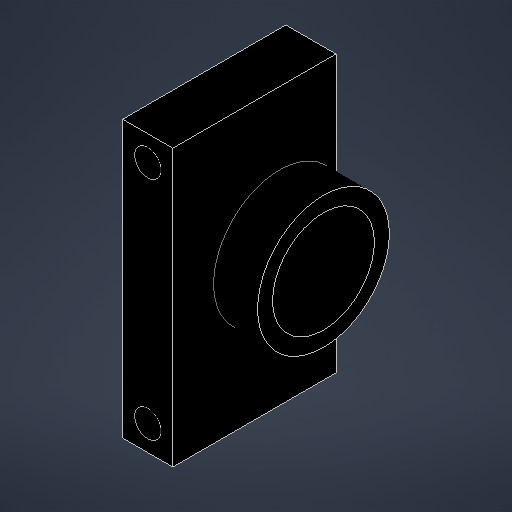
# Autodesk Inventor part: Motor Bracket
Saved by Autodesk Inventor 2026.1 (Build 301233020, 233B)
## iProperties
Created: 2025-11-06
Part Number: Motor Bracket
Material: Generic
Document SubType Name: Modeling
Designer: Bahaa
Density: 1 g/cm^3
Appearance: Black PLA
Mass: 8.44475 g
Surface Area: 48.2722 cm^2
Volume: 8.44475 cm^3
Author: Bahaa
Autodesk Inventor part; units mm, degrees
ref_plane "YZ Plane" through (0, 0, 0) normal (1, 0, 0) x (0, 1, 0)
ref_plane "XZ Plane" through (0, 0, 0) normal (0, 1, 0) x (-1, 0, 0)
sketch "Sketch1" plane through (0, 0, 0) normal (0, 1, 0) x (-1, 0, 0)
  line L0 (4, 22) -> (-4, 22)
  line L1 (-4, 22) -> (-4, -22)
  line L2 (-4, -22) -> (4, -22)
  line L3 (4, -22) -> (4, 22)
  line L4 (4, 22) -> (-4, -22) construction
  line L5 (-4, 22) -> (4, -22) construction
  point P0 (0, 0)
  dimension "d0" = 8
  dimension "d1" = 44
  constraints: 12 end point, 2 midpoint, 2 parallel, 1 horizontal, 1 perpendicular
  measures "d0" distance of L2.end L1.end
  measures "d1" distance of L1.end L0.end
extrude "Extrusion1" add sketch "Sketch1" along normal blind 26
sketch "Sketch2" plane through (4, 0, 22) normal (1, 0, 0) x (0, 0, -1)
  circle A0 centre (22, 17) radius 8.1
  line L0 (0, 0) -> (0, 26) projected
  line L1 (44, 0) -> (44, 26) projected
  line L2 (0, 0) -> (44, 0) projected
  line L3 (0, 26) -> (44, 26) projected
  circle A1 centre (22, 17) radius 4.1
  circle A2 centre (22, 17) radius 5.1
  circle A3 centre (22, 17) radius 28 construction
  circle A4 centre (22, 17) radius 10.5
  line L4 (17.7, 21.3) -> (26.3, 21.3)
  line L5 (26.3, 21.3) -> (26.3, 12.7)
  line L6 (26.3, 12.7) -> (17.7, 12.7)
  line L7 (17.7, 12.7) -> (17.7, 21.3)
  line L8 (17.7, 21.3) -> (26.3, 12.7) construction
  line L9 (26.3, 21.3) -> (17.7, 12.7) construction
  point P0 (22, 0)
  point P1 (34.4721, 0)
  point P2 (25.5279, 0)
  dimension "d4" = 16.2
  dimension "d5" = 44
  dimension "d6" = 26
  dimension "d7" = 17
  dimension "d8" = 22
  dimension "d12" = 8.2
  dimension "d15" = 10.2
  dimension "d20" = 56
  dimension "d27" = 21
  dimension "d53" = 8.6
  dimension "d54" = 8.6
  constraints: 12 end point, 5 centre point, 4 coincident, 2 midpoint, 2 parallel, 1 horizontal, 1 perpendicular
  measures "d4" diameter of A0
  measures "d5" distance between parallel lines of L0 L1
  measures "d6" distance between parallel lines of L2 L3
  measures "d7" distance from line of L2 A0.centre
  measures "d8" distance from line of L1 A0.centre
  measures "d12" diameter of A1
  measures "d15" diameter of A2
  measures "d20" diameter of A3
  measures "d27" diameter of A4
  measures "d53" distance of L5.end L6.end
  measures "d54" distance of L4.end L5.end
sketch "Sketch3" plane through (0, 26, 0) normal (0, 1, 0) x (1, 0, 0)
  line L0 (4, -22) -> (4, 22) projected
  line L1 (-4, 22) -> (-4, -22) projected
  line L2 (-4, -22) -> (4, -22) projected
  line L3 (4, 0) -> (-4, 0) construction
  point P0 (0, 0)
  point P1 (0, -18)
  point P2 (0, 18)
  dimension "d9" = 8
  dimension "d18" = 4
  dimension "d19" = 4
  constraints: 2 end point, 2 midpoint, 1 symmetric about line
  measures "d9" distance between parallel lines of L0 L1
  measures "d18" distance from line of L2 point (0, -18)
  measures "d19" distance from line of L0 point (0, -18)
extrude "Extrusion2" cut sketch "Sketch2" against normal blind 5 contours A0 | A1 | A2 L5 | L5 A2 L6 L7 L4 | A2 L4 L5 | L5 L6 A2 | L4 A2 | A2 L6 | A2 L7 L4 | L6 L7 A2 | L7 A2
extrude "Extrusion3" cut sketch "Sketch2" against normal through all contours A1 | L5 A2 L6 L7 L4 | A2 L4 L5 | L5 L6 A2 | A2 L7 L4 | L6 L7 A2
extrude "Extrusion4" cut sketch "Sketch2" against normal blind 1.15 from surface at -5 contours A2 L5 | L5 A2 L6 L7 L4 | L4 A2 | A2 L6 | L7 A2
sketch "Sketch4" plane through (-4, 0, -22) normal (-1, 0, 0) x (0, 0, 1)
  line L0 (22, 17) -> (22, 23.5) construction
  circle A0 centre (22, 23.5) radius 1.025
  circle A1 centre (16.3708, 20.25) radius 1.025
  circle A2 centre (16.3708, 13.75) radius 1.025
  circle A3 centre (22, 10.5) radius 1.025
  circle A4 centre (27.6292, 13.75) radius 1.025
  circle A5 centre (27.6292, 20.25) radius 1.025
  line L1 (0, 0) -> (0, 26) projected
  line L2 (44, 26) -> (0, 26) projected
  line L3 (44, 0) -> (0, 0) projected
  point P0 (22, 0)
  dimension "d21" = 6.5
  dimension "d22" = 2.05
  dimension "d25" = 360
  dimension "d58" = 17
  dimension "d59" = 22
  constraints: 6 centre point, 2 end point, 1 coincident, 1 vertical, 13 other
  measures "d21" distance of L0.start L0.end
  measures "d22" diameter of A0
  measures "d58" distance from line of L3 L0.start
  measures "d59" distance from line of L1 L0.start
extrude "Extrusion5" add sketch "Sketch2" along normal blind 7 contours A4 L3 | L3 A4
sketch "Sketch5" plane through (4, 0, 38) normal (1, 0, 0) x (0, 0, -1)
  circle A0 centre (38, 17) radius 10.5 projected
  line L0 (16, 0) -> (16, 26) projected
  line L1 (16, 0) -> (38, 0) projected
  line L2 (16, 26) -> (24, 26)
  line L3 (24, 26) -> (24, 0)
  line L4 (24, 0) -> (16, 0)
  line L5 (16, 0) -> (16, 26)
  line L6 (16, 26) -> (60, 26) construction
  line L7 (38, 26) -> (38, 17) construction
  line L8 (52, 26) -> (52, 0)
  line L9 (38, 0) -> (60, 0) projected
  line L10 (16, 26) -> (60, 26)
  line L11 (60, 26) -> (60, 0)
  line L12 (60, 0) -> (16, 0)
  line L13 (16, 0) -> (16, 26)
  point P0 (52, 26)
  point P1 (34.4721, 0)
  point P2 (25.5279, 0)
  point P3 (32.5917, 26)
  point P4 (43.4083, 26)
  dimension "d30" = 8
  constraints: 20 end point, 4 parallel, 2 horizontal, 2 perpendicular, 2 symmetric about line, 1 midpoint, 1 point on line, 1 vertical, 1 other
  measures "d30" distance of L3.end L4.end
extrude "Extrusion6" [suppressed]
fillet "Fillet1" [suppressed]
hole "Hole1" at (0, 26, 18) at (0, 26, -18) direction (0, -1, 0) diameter 4.2 depth 6
ref_plane "Work Plane1" through (0, 13, 0) normal (0, 1, 0) x (1, 0, 0)
mirror "Mirror1" about plane through (0, 13, 0) normal (0, 1, 0) of "Hole1"
hole "Hole2" at (-4, 23.5, 0) at (-4, 20.25, 5.6292) at (-4, 13.75, 5.6292) at (-4, 10.5, 0) at (-4, 13.75, -5.6292) at (-4, 20.25, -5.6292) direction (1, 0, 0) diameter 2.2 end through all countersink diameter 4.4 countersink angle 90 clearance for "Countersunk Flat Head Screw ISO 2009/7046" size "M2" standard "ISO"
extrude "Extrusion8" [suppressed]
fillet "Fillet3" radius 2 4 edges at (-2.2469, 21.3, 4.3) (-2.2469, 12.7, 4.3) (-2.2469, 21.3, -4.3) (-2.2469, 12.7, -4.3)
equation "\"d8\" = 0.5 * d5"
equation "\"d19\" = 0.5 * d9"
equation "\"d30\" = 2 * d18"
body "Solid1"
